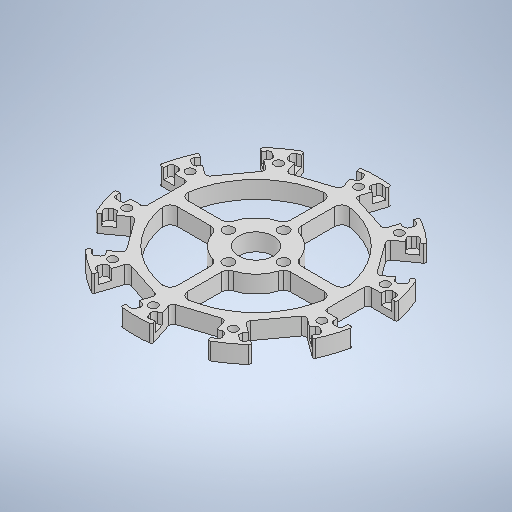
# Autodesk Inventor part: T5.0_base1
Saved by Autodesk Inventor 2025 (Build 290162000, 162)
## iProperties
Created: 2024-06-25
Part Number: T5.0_base1
Material: 一般
Document SubType Name: Modeling
Designer: 8326d
Density: 1 g/cm^3
Appearance: 既定
Author: 8326d
Autodesk Inventor part; units mm, degrees
ref_plane "YZ Plane" through (0, 0, 0) normal (1, 0, 0) x (0, 1, 0)
ref_plane "XZ Plane" through (0, 0, 0) normal (0, 1, 0) x (-1, 0, 0)
ref_plane "XY Plane" through (0, 0, 0) normal (0, 0, 1) x (1, 0, 0)
sketch "スケッチ1" plane through (0, 0, 0) normal (0, 1, 0) x (-1, 0, 0)
  circle A0 centre (0, 0) radius 35
  dimension "d0" = 70
  constraints: 1 centre point, 1 coincident
  measures "d0" diameter of A0
extrude "押し出し1" add sketch "スケッチ1" along normal blind 5
sketch "スケッチ2" plane through (0, 5, 0) normal (0, 1, 0) x (1, 0, 0)
  circle A0 centre (0, 0) radius 35 projected
  line L0 (-29.975, -8.5) -> (-33.025, -8.5)
  line L1 (-33.025, -8.5) -> (-33.025, 8.5)
  line L2 (-33.025, 8.5) -> (-29.975, 8.5)
  line L3 (-29.975, 8.5) -> (-29.975, -8.5)
  line L4 (-29.975, -8.5) -> (-33.025, 8.5) construction
  line L5 (-33.025, -8.5) -> (-29.975, 8.5) construction
  line L6 (-26, -6.3443) -> (-37, -6.3443)
  line L7 (-37, -6.3443) -> (-37, 6.3443)
  line L8 (-37, 6.3443) -> (-26, 6.3443)
  line L9 (-26, 6.3443) -> (-26, -6.3443)
  line L10 (-26, -6.3443) -> (-37, 6.3443) construction
  line L11 (-37, -6.3443) -> (-26, 6.3443) construction
  line L12 (-37, -6.3443) -> (0, 0) construction
  line L13 (0, 0) -> (-35, 0) construction
  point P0 (-31.5, 0)
  point P1 (-33.025, 6.3443)
  point P2 (-34.4202, 6.3443)
  point P3 (-34.4202, -6.3443)
  point P4 (-33.025, -6.3443)
  point P5 (-29.975, -6.3443)
  point P6 (-29.975, 6.3443)
  dimension "d3" = 31.5
  dimension "d4" = 17
  dimension "d5" = 3.05
  dimension "d6" = 9.73
  dimension "d7" = 2
  constraints: 28 end point, 4 midpoint, 4 parallel, 3 horizontal, 2 perpendicular, 1 horizontal alignment, 2 other
  measures "d3" distance of point (0, 0) point (-31.5, 0)
  measures "d4" distance of L0.end L1.end
  measures "d5" distance between parallel lines of L3 L1
  measures "d6" angle of L13 L12
  measures "d7" distance from line of L13.end L7
extrude "押し出し2" cut sketch "スケッチ2" against normal blind 3.05 contours L8 L3 L6 L1 | L1 L2 L3 L8 | L6 L3 L0 L1
extrude "押し出し3" cut sketch "スケッチ2" against normal through all contours L8 L1 L6 A0 | A0 L6 L7 L8 | L8 L3 L6 L1 | L8 L9 L6 L3
fillet "フィレット1" radius 1 6 edges at (-33.025, 3.475, -8.5) (-29.975, 3.475, -8.5) (-29.975, 3.475, 8.5) (-33.025, 3.475, 8.5) (-26, 2.5, 6.3443) (-26, 2.5, -6.3443)
pattern_circular "円形状パターン1" count 10 over 360 about axis through (0, -10, 0) along (0, 1, 0) of "押し出し2", "押し出し3", "フィレット1"
sketch "スケッチ3" plane through (0, 5, 0) normal (0, 1, 0) x (1, 0, 0)
  point P0 (0, 0)
  point P1 (0, -29.75)
  dimension "d16" = 29.75
  constraints: 1 vertical alignment
  measures "d16" distance of point (0, 0) point (0, -29.75)
hole "穴1" at (0, 5, 29.75) direction (0, -1, 0) diameter 2.5 end through all
pattern_circular "円形状パターン2" count 10 over 360 about axis through (0, -10, 0) along (0, 1, 0) of "穴1"
fillet "フィレット3" radius 0.5 20 edges at (4.6027, 2.5, 34.696) (-4.6027, 2.5, 34.696) (-16.6702, 2.5, 30.7751) (-24.1174, 2.5, 25.3643) (-31.5756, 2.5, 15.099) (-34.4202, 2.5, 6.3443) (-34.4202, 2.5, -6.3443) (-31.5756, 2.5, -15.099) (-24.1174, 2.5, -25.3643) (-16.6702, 2.5, -30.7751) (-4.6027, 2.5, -34.696) (4.6027, 2.5, -34.696) (16.6702, 2.5, -30.7751) (24.1174, 2.5, -25.3643) (31.5756, 2.5, -15.099) (34.4202, 2.5, -6.3443) (34.4202, 2.5, 6.3443) (31.5756, 2.5, 15.099) (24.1174, 2.5, 25.3643) (16.6702, 2.5, 30.7751)
sketch "スケッチ4" plane through (0, 5, 0) normal (0, 1, 0) x (1, 0, 0)
  circle A0 centre (0, 0) radius 23.625
  circle A1 centre (0, 0) radius 10
  line L0 (-1.5, 9.8869) -> (-1.5, 23.5773)
  line L1 (0, 0) -> (-23.625, 0) construction
  line L2 (0, 0) -> (23.625, 0) construction
  line L3 (-9.8869, 1.5) -> (-23.5773, 1.5)
  circle A2 centre (0, 8) radius 3
  circle A3 centre (-8, 0) radius 3
  point P0 (-10.5981, 1.5)
  point P1 (-9.6875, 2.4804)
  point P2 (-2.4804, 9.6875)
  point P3 (-1.5, 10.5981)
  dimension "d29" = 47.25
  dimension "d30" = 20
  dimension "d31" = 180
  dimension "d32" = 1.5
  dimension "d33" = 1.5
  dimension "d43" = 6
  dimension "d44" = 6
  dimension "d45" = 8
  dimension "d46" = 8
  constraints: 8 end point, 5 point on circle, 4 centre point, 2 coincident, 1 collinear, 1 horizontal, 1 parallel, 1 point on line, 1 vertical, 1 vertical alignment
  measures "d29" diameter of A0
  measures "d30" diameter of A1
  measures "d31" angle of L1 L2
  measures "d32" distance from line of point (0, 0) L0
  measures "d33" distance between parallel lines of L1 L3
  measures "d43" diameter of A2
  measures "d44" diameter of A3
  measures "d45" distance of point (0, 0) A2.centre
  measures "d46" distance of point (0, 0) A3.centre
extrude "押し出し4" cut sketch "スケッチ4" against normal through all contours L0 A2 A1 A3 L3 A0 picked at (-17.2286, 7.9329)
fillet "フィレット4" radius 2 6 edges at (-23.5773, 2.5, -1.5) (-1.5, 2.5, -23.5773) (-10.5981, 2.5, -1.5) (-9.6875, 2.5, -2.4804) (-2.4804, 2.5, -9.6875) (-1.5, 2.5, -10.5981)
pattern_circular "円形状パターン3" count 4 over 360 about axis through (0, -10, 0) along (0, 1, 0) of "押し出し4", "フィレット4"
sketch "スケッチ5" plane through (0, 5, 0) normal (0, 1, 0) x (1, 0, 0)
  circle A0 centre (0, 0) radius 5.05
  dimension "d40" = 10.1
  constraints: 1 centre point, 1 coincident
  measures "d40" diameter of A0
extrude "押し出し5" cut sketch "スケッチ5" against normal through all
sketch "スケッチ6" plane through (0, 5, 0) normal (0, 1, 0) x (1, 0, 0)
  arc A0 (-2.1, 10.1424) -> (-2.1786, 10.0625) centre (0, 8) ccw projected
  arc A1 (-10.0625, 2.1786) -> (-10.1424, 2.1) centre (-8, 0) ccw projected
  arc A2 (-2.1786, -10.0625) -> (-2.1, -10.1424) centre (0, -8) ccw projected
  arc A3 (10.0625, -2.1786) -> (10.1424, -2.1) centre (8, 0) ccw projected
  point P0 (0, 0)
hole "穴2" at (0, 5, -8) at (-8, 5, 0) at (0, 5, 8) at (8, 5, 0) direction (0, -1, 0) diameter 3.1 end through all
equation "\"d0\" = 2 * r"
equation "\"d3\" = 0.9 * r"
equation "\"d16\" = 0.85 * r"
equation "\"d29\" = 1.35 * r"
equation "\"d33\" = d32"
equation "\"d46\" = d45"
equation "\"r\" = 35"
